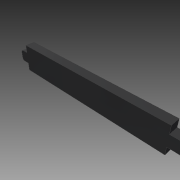
# Autodesk Inventor part: spool_stand_brace_top
Saved by Autodesk Inventor 2014 (Build 180170000, 170)
## iProperties
Created: 2014-04-08
Part Number: spool_stand_brace_top
Material: Plywood, Finish
Document SubType Name: Modeling
Designer: buben
Density: 0.552 g/cm^3
Appearance: Plywood - New
Author: buben
Autodesk Inventor part; units mm, degrees
ref_plane "YZ Plane" through (0, 0, 0) normal (1, 0, 0) x (0, 1, 0)
ref_plane "XZ Plane" through (0, 0, 0) normal (0, 1, 0) x (-1, 0, 0)
ref_plane "XY Plane" through (0, 0, 0) normal (0, 0, 1) x (1, 0, 0)
sketch "Sketch1" plane through (0, 0, 0) normal (0, 1, 0) x (-1, 0, 0)
  line L0 (0, 0) -> (-110, 0)
  line L1 (-110, 0) -> (-110, -18.805)
  line L2 (-110, -18.805) -> (0, -18.805)
  line L3 (0, -18.805) -> (0, 0)
  dimension "d0" = 110
  dimension "d1" = 18.805
  constraints: 8 end point, 2 parallel, 1 horizontal, 1 perpendicular
  measures "d0" distance of L0.start L0.end
  measures "d1" distance of L2.end L0.start
extrude "Extrusion1" add sketch "Sketch1" along normal blind 6.5
sketch "Sketch2" plane through (0, 6.5, 0) normal (0, 1, 0) x (1, 0, 0)
  line L0 (110, 0) -> (110, 18.805) projected
  line L1 (0, 18.805) -> (0, 0) projected
  line L2 (0, 13.4025) -> (-4.5, 13.4025)
  line L3 (-6.5, 11.4025) -> (-6.5, 7.4025)
  line L4 (-4.5, 5.4025) -> (0, 5.4025)
  line L5 (0, 5.4025) -> (0, 13.4025)
  line L6 (110, 13.4025) -> (117.5, 13.4025)
  line L7 (119.5, 11.4025) -> (119.5, 7.4025)
  line L8 (117.5, 5.4025) -> (110, 5.4025)
  line L9 (110, 5.4025) -> (110, 13.4025)
  arc A0 (-4.5, 13.4025) -> (-6.5, 11.4025) centre (-4.5, 11.4025) ccw
  arc A1 (-6.5, 7.4025) -> (-4.5, 5.4025) centre (-4.5, 7.4025) ccw
  arc A2 (119.5, 11.4025) -> (117.5, 13.4025) centre (117.5, 11.4025) ccw
  arc A3 (117.5, 5.4025) -> (119.5, 7.4025) centre (117.5, 7.4025) ccw
  point P0 (-6.5, 9.4025)
  point P1 (0, 9.4025)
  dimension "d4" = 2
  dimension "d5" = 8
  dimension "d6" = 6.5
  dimension "d7" = 9.5
  constraints: 16 end point, 8 point on circle, 8 tangent, 4 centre point, 4 parallel, 3 equal radius, 2 collinear, 2 horizontal, 2 midpoint, 2 perpendicular, 2 point on line, 1 horizontal alignment
  measures "d4" radius of A0
  measures "d5" distance between parallel lines of L4 L2
  measures "d6" distance between parallel lines of L1 L3
  measures "d7" distance between parallel lines of L9 L7
extrude "Extrusion2" add sketch "Sketch2" against normal blind 6.5
body "Solid1"
